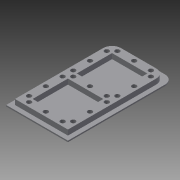
# Autodesk Inventor part: edition 2
Saved by Autodesk Inventor 2015 (Build 190159000, 159)
## iProperties
Created: 2015-03-23
Part Number: edition 2
Material: Generic
Document SubType Name: Modeling
Designer: Jason
Density: 1 g/cm^3
Appearance: Default
Author: Jason
Autodesk Inventor part; units mm, degrees
ref_plane "YZ Plane" through (0, 0, 0) normal (1, 0, 0) x (0, 1, 0)
ref_plane "XZ Plane" through (0, 0, 0) normal (0, 1, 0) x (-1, 0, 0)
ref_plane "XY Plane" through (0, 0, 0) normal (0, 0, 1) x (1, 0, 0)
sketch "Sketch1" plane through (0, 0, 0) normal (0, 0, 1) x (1, 0, 0)
  line L0 (0, 0) -> (70, 0)
  line L1 (70, 0) -> (70, -120)
  line L2 (70, -120) -> (0, -120)
  line L3 (0, -120) -> (0, 0)
  dimension "d0" = 70
  dimension "d1" = 120
  constraints: 8 end point, 2 parallel, 1 horizontal, 1 perpendicular
  measures "d0" distance of L1.end L2.end
  measures "d1" distance of L0.end L1.end
extrude "Extrusion1" add sketch "Sketch1" along normal blind 7.4
sketch "Sketch2" plane through (0, 0, 7.4) normal (0, 0, 1) x (1, 0, 0)
  circle A0 centre (10, -104) radius 2.6
  circle A1 centre (16, -110) radius 2.6
  circle A2 centre (35, -110) radius 2.6
  circle A3 centre (10, -66) radius 2.6
  circle A4 centre (16, -60) radius 2.6
  circle A5 centre (10, -35) radius 2.6
  circle A6 centre (10, -16) radius 2.6
  circle A7 centre (16, -10) radius 2.6
  circle A8 centre (35, -60) radius 2.6
  circle A9 centre (60, -104) radius 2.6
  circle A10 centre (60, -66) radius 2.6
  circle A11 centre (10, -85) radius 2.6
  circle A12 centre (60, -85) radius 2.6
  circle A13 centre (54, -110) radius 2.6
  circle A14 centre (54, -60) radius 2.6
  circle A15 centre (60, -54) radius 2.6
  circle A16 centre (60, -16) radius 2.6
  circle A17 centre (10, -54) radius 2.6
  circle A18 centre (35, -10) radius 2.6
  circle A19 centre (54, -10) radius 2.6
  line L0 (0, 0) -> (0, -120) projected
  line L1 (70, -120) -> (70, 0) projected
  line L2 (70, 0) -> (0, 0) projected
  line L3 (0, -120) -> (70, -120) projected
  circle A20 centre (60, -35) radius 2.6
  dimension "d5" = 5.2
  dimension "d6" = 5.2
  dimension "d7" = 5.2
  dimension "d10" = 5.2
  dimension "d11" = 5.2
  dimension "d12" = 5.2
  dimension "d15" = 5.2
  dimension "d16" = 5.2
  dimension "d17" = 5.2
  dimension "d19" = 5.2
  dimension "d20" = 5.2
  dimension "d21" = 5.2
  dimension "d22" = 5.2
  dimension "d23" = 5.2
  dimension "d24" = 5.2
  dimension "d25" = 5.2
  dimension "d26" = 5.2
  dimension "d27" = 5.2
  dimension "d54" = 10
  dimension "d55" = 10
  dimension "d56" = 16
  dimension "d57" = 16
  dimension "d58" = 16
  dimension "d59" = 35
  dimension "d60" = 10
  dimension "d61" = 19
  dimension "d62" = 19
  dimension "d63" = 19
  dimension "d64" = 5.2
  dimension "d67" = 6
  dimension "d68" = 6
  dimension "d69" = 6
  dimension "d70" = 6
  dimension "d71" = 19
  dimension "d72" = 19
  dimension "d74" = 6
  dimension "d75" = 10
  constraints: 21 centre point
  measures "d5" diameter of A0
  measures "d6" diameter of A1
  measures "d7" diameter of A2
  measures "d10" diameter of A3
  measures "d11" diameter of A4
  measures "d12" diameter of A5
  measures "d15" diameter of A7
  measures "d16" diameter of A8
  measures "d17" diameter of A9
  measures "d19" diameter of A11
  measures "d20" diameter of A12
  measures "d21" diameter of A13
  measures "d22" diameter of A14
  measures "d23" diameter of A15
  measures "d24" diameter of A16
  measures "d25" diameter of A17
  measures "d26" diameter of A18
  measures "d27" diameter of A19
  measures "d54" distance from line of L2 A7.centre
  measures "d55" distance from line of L0 A6.centre
  measures "d56" distance from line of L0 A7.centre
  measures "d57" distance from line of L2 A6.centre
  measures "d58" distance from line of L1 A19.centre
  measures "d59" distance from line of L1 A18.centre
  measures "d60" distance from line of L1 A16.centre
  measures "d61" distance of A19.centre A18.centre
  measures "d62" distance of A5.centre A6.centre
  measures "d63" distance of A17.centre A5.centre
  measures "d64" diameter of A20
  measures "d67" horizontal distance of A4.centre A17.centre
  measures "d68" horizontal distance of A4.centre A17.centre
  measures "d69" horizontal distance of A4.centre A3.centre
  measures "d70" horizontal distance of A10.centre A14.centre
  measures "d71" distance of A11.centre A3.centre
  measures "d72" distance of A0.centre A11.centre
  measures "d74" horizontal distance of A1.centre A0.centre
  measures "d75" distance from line of L3 A1.centre
extrude "Extrusion2" cut sketch "Sketch2" against normal through all contours A0 | A1 | A2 | A3 | A4 | A5 | A6 | A7 | A8 | A9 | A10 | A11 | A12 | A13 | A14 | A15 | A16 | A17 | A18 | A19 | A20
sketch "Sketch3" plane through (0, 0, 7.4) normal (0, 0, 1) x (1, 0, 0)
  line L0 (15, -15) -> (55, -15)
  line L1 (55, -15) -> (55, -55)
  line L2 (55, -55) -> (15, -55)
  line L3 (15, -55) -> (15, -15)
  line L4 (15, -65) -> (55, -65)
  line L5 (55, -65) -> (55, -105)
  line L6 (55, -105) -> (15, -105)
  line L7 (15, -105) -> (15, -65)
  line L8 (0, 0) -> (0, -120) projected
  line L9 (70, 0) -> (0, 0) projected
  line L10 (0, -120) -> (70, -120) projected
  line L11 (70, -120) -> (70, 0) projected
  circle A0 centre (35, -10) radius 2.6 projected
  circle A1 centre (35, -60) radius 2.6 projected
  line L12 (5, -5) -> (65, -5)
  line L13 (65, -5) -> (65, -115)
  line L14 (65, -115) -> (5, -115)
  line L15 (5, -115) -> (5, -5)
  circle A2 centre (16, -10) radius 2.6 projected
  circle A3 centre (60, -16) radius 2.6 projected
  circle A4 centre (10, -35) radius 2.6 projected
  circle A5 centre (35, -110) radius 2.6 projected
  dimension "d47" = 15
  dimension "d48" = 15
  dimension "d76" = 15
  dimension "d77" = 15
  dimension "d78" = 15
  dimension "d80" = 5
  dimension "d81" = 5
  dimension "d82" = 5
  dimension "d83" = 5
  dimension "d84" = 5
  dimension "d85" = 5
  constraints: 24 end point, 6 parallel, 3 horizontal, 3 perpendicular, 1 point on line
  measures "d47" distance between parallel lines of L3 L8
  measures "d48" distance between parallel lines of L9 L0
  measures "d76" distance between parallel lines of L11 L1
  measures "d77" distance between parallel lines of L11 L5
  measures "d78" distance between parallel lines of L10 L6
  measures "d80" distance from line of A1.centre L2
  measures "d81" distance from line of A1.centre L4
  measures "d82" distance from line of A2.centre L12
  measures "d83" distance from line of A3.centre L13
  measures "d84" distance from line of A4.centre L15
  measures "d85" distance from line of A5.centre L14
extrude "Extrusion3" cut sketch "Sketch3" against normal blind 5.9 contours L0 L1 L2 L3 | L4 L5 L6 L7 | L9 L11 L10 L8
fillet "Fillet1" radius 10 2 edges at (70, 0, 0.75) (0, 0, 0.75)
fillet "Fillet2" radius 10 2 edges at (65, -5, 4.45) (5, -5, 4.45)
body "Solid1"
